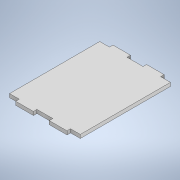
# Autodesk Inventor part: backstop_beslag
Saved by Autodesk Inventor 2022 (Build 260153000, 153)
## iProperties
Created: 2022-04-28
Part Number: backstop_beslag
Material: Generic
Document SubType Name: Sheet Metal
Designer: patri
Density: 1 g/cm^3
Sheet Metal Rule: Default_mm
Appearance: Default
Author: patri
Autodesk Inventor part; units mm, degrees
ref_plane "YZ Plane" through (0, 0, 0) normal (1, 0, 0) x (0, 1, 0)
ref_plane "XZ Plane" through (0, 0, 0) normal (0, 1, 0) x (-1, 0, 0)
ref_plane "XY Plane" through (0, 0, 0) normal (0, 0, 1) x (1, 0, 0)
sketch "Sketch1" plane through (0, 0, 0) normal (0, 1, 0) x (-1, 0, 0)
  line L0 (40, 0) -> (34.5, 0)
  line L1 (34.5, 0) -> (34.5, 2)
  line L2 (34.5, 2) -> (24.5, 2)
  line L3 (24.5, 2) -> (24.5, 0)
  line L4 (24.5, 0) -> (15.5, 0)
  line L5 (15.5, 0) -> (15.5, 2)
  line L6 (15.5, 2) -> (5.5, 2)
  line L7 (5.5, 2) -> (5.5, 0)
  line L8 (5.5, 0) -> (0, 0)
  line L9 (0, 0) -> (0, -25.5)
  line L10 (0, -25.5) -> (40, -25.5)
  line L11 (40, -25.5) -> (40, 0)
  line L12 (40, -51) -> (34.5, -51)
  line L13 (34.5, -51) -> (34.5, -53)
  line L14 (34.5, -53) -> (24.5, -53)
  line L15 (24.5, -53) -> (24.5, -51)
  line L16 (24.5, -51) -> (15.5, -51)
  line L17 (15.5, -51) -> (15.5, -53)
  line L18 (15.5, -53) -> (5.5, -53)
  line L19 (5.5, -53) -> (5.5, -51)
  line L20 (5.5, -51) -> (0, -51)
  line L21 (0, -51) -> (0, -25.5)
  line L22 (40, -25.5) -> (40, -51)
  dimension "d1" = 40
  dimension "d2" = 10
  dimension "d3" = 10
  dimension "d4" = 5.5
  dimension "d5" = 5.5
  dimension "d6" = 2
  dimension "d7" = 25.5
  measures "d1" distance of L9.end L10.end
  measures "d2" distance of L1.end L2.end
  measures "d3" distance of L5.end L6.end
  measures "d4" distance between parallel lines of L9 L7
  measures "d5" distance between parallel lines of L11 L1
  measures "d6" distance of L0.end L1.end
  measures "d7" distance of L10.end L0.start
extrude "Plate1" add sketch "Sketch1" along normal blind 2
equation "\"d8\" = Thickness"
equation "\"BendRadius\" = Thickness"
equation "\"BendReliefWidth\" = Thickness"
equation "\"BendReliefDepth\" = 0.5 * Thickness"
equation "\"CornerReliefSize\" = 4 * Thickness"
equation "\"MinimumRemnant\" = 2 * Thickness"
equation "\"TransitionRadius\" = BendRadius"
equation "\"JacobiRadiusSize\" = BendRadius"
equation "\"GapSize\" = Thickness"
equation "\"Thickness\" = 2"
body "Solid1"
